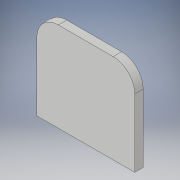
# Autodesk Inventor part: Encoder
Saved by Autodesk Inventor 2019.3 (Build 233278000, 278)
## iProperties
Created: 2020-02-04
Part Number: Encoder
Material: Типовые
Document SubType Name: Modeling
Designer: ШП
Density: 1 g/cm^3
Appearance: По умолчанию
Author: ШП
Autodesk Inventor part; units mm, degrees
ref_plane "YZ Plane" through (0, 0, 0) normal (1, 0, 0) x (0, 1, 0)
ref_plane "XZ Plane" through (0, 0, 0) normal (0, 1, 0) x (-1, 0, 0)
ref_plane "XY Plane" through (0, 0, 0) normal (0, 0, 1) x (1, 0, 0)
sketch "Эскиз1" plane through (0, 0, 0) normal (0, 0, 1) x (1, 0, 0)
  line L0 (0, 0) -> (11.6, 0)
  line L1 (11.6, 0) -> (11.6, 10.6)
  line L2 (11.6, 10.6) -> (0, 10.6)
  line L3 (0, 10.6) -> (0, 0)
  dimension "d0" = 11.6
  dimension "d1" = 10.6
  constraints: 8 end point, 2 parallel, 1 horizontal, 1 perpendicular
  measures "d0" distance of L2.end L1.end
  measures "d1" distance of L1.end L0.end
extrude "Выдавливание1" add sketch "Эскиз1" along normal blind 1
fillet "Сопряжение1" radius 2.55 2 edges at (11.6, 10.6, 0.5) (0, 10.6, 0.5)
